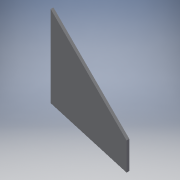
# Autodesk Inventor part: Aleta2
Saved by Autodesk Inventor 2019.4 (Build 234330000, 330)
## iProperties
Created: 2022-01-21
Part Number: Aleta2
Material: Generic
Document SubType Name: Modeling
Designer: juand
Density: 1 g/cm^3
Appearance: Default
Author: juand
Autodesk Inventor part; units mm, degrees
ref_plane "YZ Plane" through (0, 0, 0) normal (1, 0, 0) x (0, 1, 0)
ref_plane "XZ Plane" through (0, 0, 0) normal (0, 1, 0) x (-1, 0, 0)
ref_plane "XY Plane" through (0, 0, 0) normal (0, 0, 1) x (1, 0, 0)
sketch "Sketch1" plane through (0, 0, 0) normal (0, 0, 1) x (1, 0, 0)
  line L0 (-82, 112) -> (0, 30)
  line L1 (-82, 112) -> (-82, 24)
  line L2 (-82, 112) -> (-82, 24)
  line L3 (-82, 24) -> (0, 0)
  line L4 (0, 30) -> (0, 0)
  line L5 (0, 0) -> (0, 30)
  line L6 (0, 30) -> (-82, 112)
  constraints: 14 end point, 1 collinear, 1 vertical
extrude "Extrusion1" add sketch "Sketch1" along normal blind 3
body "Solid1"
